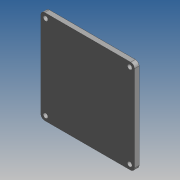
# Autodesk Inventor part: P035_FondBoitierv3
Saved by Autodesk Inventor 2021.3 (Build 253353000, 353)
## iProperties
Created: 2021-11-26
Part Number: P035_FondBoitierv3
Material: Générique
Document SubType Name: Modeling
Designer: gabri
Density: 1 g/cm^3
Appearance: Par défaut
Author: gabri
Autodesk Inventor part; units mm, degrees
ref_plane "YZ Plane" through (0, 0, 0) normal (1, 0, 0) x (0, 1, 0)
ref_plane "XZ Plane" through (0, 0, 0) normal (0, 1, 0) x (-1, 0, 0)
ref_plane "XY Plane" through (0, 0, 0) normal (0, 0, 1) x (1, 0, 0)
sketch "Sketch2" plane through (0, 0, 0) normal (0, 1, 0) x (-1, 0, 0)
  line L0 (-46, -50) -> (46, -50)
  line L1 (50, -46) -> (50, 46)
  line L2 (46, 50) -> (-46, 50)
  line L3 (-50, 46) -> (-50, -46)
  line L4 (-50, -50) -> (50, 50) construction
  line L5 (50, -50) -> (-50, 50) construction
  arc A0 (50, 46) -> (46, 50) centre (46, 46) ccw
  arc A1 (-46, 50) -> (-50, 46) centre (-46, 46) ccw
  arc A2 (-50, -46) -> (-46, -50) centre (-46, -46) ccw
  arc A3 (46, -50) -> (50, -46) centre (46, -46) ccw
  point P0 (0, 0)
  dimension "d0" = 100
  dimension "d1" = 100
  dimension "d4" = 4
  dimension "d5" = 4
  constraints: 12 end point, 8 point on circle, 8 point on line, 8 tangent, 4 centre point, 2 equal radius, 2 midpoint, 2 parallel, 1 horizontal, 1 perpendicular
  measures "d0" distance of L5.end L4.end
  measures "d1" distance between parallel lines of L0 L2
  measures "d4" radius of A0
  measures "d5" radius of A1
extrude "Extrusion1" add sketch "Sketch2" along normal blind 5
sketch "Sketch3" plane through (0, 0, 0) normal (0, -1, 0) x (1, 0, 0)
  arc A0 (-50, -46) -> (-46, -50) centre (-46, -46) ccw construction
  line L0 (46, -50) -> (-46, -50) construction
  arc A1 (46, -50) -> (50, -46) centre (46, -46) ccw construction
  line L1 (50, 46) -> (50, -46) construction
  arc A2 (50, 46) -> (46, 50) centre (46, 46) ccw construction
  line L2 (-46, 50) -> (46, 50) construction
  arc A3 (-46, 50) -> (-50, 46) centre (-46, 46) ccw construction
  line L3 (-50, -46) -> (-50, 46) construction
  point P0 (0, 0)
  point P1 (-45, 45)
  point P2 (45, 45)
  point P3 (-45, -45)
  point P4 (45, -45)
  dimension "d13" = 5
  dimension "d14" = 5
  dimension "d17" = 90
  dimension "d20" = 90
  constraints: 1 horizontal, 1 vertical, 3 other
  measures "d13" distance from line of L2 point (-45, 45)
  measures "d14" distance from line of L3 point (-45, 45)
  measures "d17" distance of point (-45, 45) point (45, 45)
  measures "d20" distance of point (-45, 45) point (-45, -45)
hole "Hole1" at (-45, 0, 45) at (45, 0, 45) at (45, 0, -45) at (-45, 0, -45) direction (0, 1, 0) diameter 5 depth 14.2 tip angle 118
sketch "Sketch4" plane through (0, 5, 0) normal (0, 1, 0) x (1, 0, 0)
  circle A0 centre (45, 45) radius 2.5 construction
  circle A1 centre (-45, -45) radius 2.5 construction
  circle A2 centre (45, -45) radius 2.5 construction
  circle A3 centre (-45, 45) radius 2.5 construction
  arc A4 (-46, 50) -> (-50, 46) centre (-46, 46) ccw construction
  line L0 (-50, 46) -> (-50, -46) construction
  arc A5 (-50, -46) -> (-46, -50) centre (-46, -46) ccw construction
  line L1 (-46, -50) -> (46, -50) construction
  arc A6 (46, -50) -> (50, -46) centre (46, -46) ccw construction
  line L2 (50, -46) -> (50, 46) construction
  arc A7 (50, 46) -> (46, 50) centre (46, 46) ccw construction
  line L3 (46, 50) -> (-46, 50) construction
  arc A8 (44.6333, -39.5122) -> (39.5122, -44.6333) centre (45, -45) ccw
  arc A9 (45.9545, -41.6327) -> (41.6327, -45.9545) centre (45, -45) ccw
  line L4 (39.7085, -48.5) -> (-39.7085, -48.5)
  line L5 (48.5, -39.7085) -> (48.5, 39.7085)
  line L6 (46.5, -37.5167) -> (46.5, 37.5167)
  line L7 (0, -72.209) -> (0, 64.6676) construction
  line L8 (107.9328, 0) -> (-102.5907, 0) construction
  line L9 (37.5167, -46.5) -> (-37.5167, -46.5)
  arc A10 (-39.5122, -44.6333) -> (-44.6333, -39.5122) centre (-45, -45) ccw
  arc A11 (-41.6327, -45.9545) -> (-45.9545, -41.6327) centre (-45, -45) ccw
  line L10 (-48.5, -39.7085) -> (-48.5, 39.7085)
  line L11 (-46.5, 37.5167) -> (-46.5, -37.5167)
  arc A12 (41.6327, 45.9545) -> (45.9545, 41.6327) centre (45, 45) ccw
  arc A13 (39.5122, 44.6333) -> (44.6333, 39.5122) centre (45, 45) ccw
  line L12 (39.7085, 48.5) -> (-39.7085, 48.5)
  line L13 (37.5167, 46.5) -> (-37.5167, 46.5)
  line L14 (46, 50) -> (-46, 50) construction
  arc A14 (-44.6333, 39.5122) -> (-39.5122, 44.6333) centre (-45, 45) ccw
  arc A15 (-45.9545, 41.6327) -> (-41.6327, 45.9545) centre (-45, 45) ccw
  arc A16 (39.7085, -48.5) -> (41.6327, -45.9545) centre (39.7085, -46.5) ccw
  arc A17 (37.5167, -46.5) -> (39.5122, -44.6333) centre (37.5167, -44.5) ccw
  arc A18 (45.9545, -41.6327) -> (48.5, -39.7085) centre (46.5, -39.7085) ccw
  arc A19 (44.6333, -39.5122) -> (46.5, -37.5167) centre (44.5, -37.5167) ccw
  arc A20 (-41.6327, -45.9545) -> (-39.7085, -48.5) centre (-39.7085, -46.5) ccw
  arc A21 (-39.5122, -44.6333) -> (-37.5167, -46.5) centre (-37.5167, -44.5) ccw
  arc A22 (-48.5, -39.7085) -> (-45.9545, -41.6327) centre (-46.5, -39.7085) ccw
  arc A23 (-46.5, -37.5167) -> (-44.6333, -39.5122) centre (-44.5, -37.5167) ccw
  arc A24 (-44.6333, 39.5122) -> (-46.5, 37.5167) centre (-44.5, 37.5167) ccw
  arc A25 (-45.9545, 41.6327) -> (-48.5, 39.7085) centre (-46.5, 39.7085) ccw
  arc A26 (-39.7085, 48.5) -> (-41.6327, 45.9545) centre (-39.7085, 46.5) ccw
  arc A27 (-37.5167, 46.5) -> (-39.5122, 44.6333) centre (-37.5167, 44.5) ccw
  arc A28 (41.6327, 45.9545) -> (39.7085, 48.5) centre (39.7085, 46.5) ccw
  arc A29 (39.5122, 44.6333) -> (37.5167, 46.5) centre (37.5167, 44.5) ccw
  arc A30 (48.5, 39.7085) -> (45.9545, 41.6327) centre (46.5, 39.7085) ccw
  arc A31 (46.5, 37.5167) -> (44.6333, 39.5122) centre (44.5, 37.5167) ccw
  point P0 (0, 0)
  point P1 (45, -48.5)
  point P2 (39.7085, -46.5)
  point P3 (48.5, -45)
  point P4 (48.5, 45)
  point P5 (46.5, -39.7085)
  point P6 (46.5, 39.7085)
  point P7 (-45, -48.5)
  point P8 (-48.5, -45)
  point P9 (-46.5, 39.7085)
  point P10 (-46.5, -39.7085)
  point P11 (45, 48.5)
  point P12 (-45, 48.5)
  point P13 (39.7085, 46.5)
  point P14 (-39.7085, 46.5)
  point P15 (-48.5, 45)
  dimension "d23" = 5.5
  dimension "d24" = 3.5
  dimension "d25" = 1.5
  dimension "d27" = 1.5
  dimension "d28" = 2
  dimension "d31" = 5.5
  dimension "d32" = 3.5
  dimension "d33" = 2
  dimension "d34" = 1.5
  dimension "d35" = 2
  dimension "d36" = 5.5
  dimension "d37" = 3.5
  dimension "d38" = 1.5
  dimension "d39" = 2
  dimension "d41" = 5.5
  dimension "d42" = 3.5
  dimension "d43" = 2
  dimension "d44" = 2
  dimension "d45" = 2
  constraints: 64 point on circle, 32 tangent, 24 centre point, 20 end point, 16 point on line, 13 equal radius, 8 coincident, 6 parallel, 4 horizontal, 1 vertical
  measures "d23" radius of A8
  measures "d24" radius of A9
  measures "d25" distance between parallel lines of L1 L4
  measures "d27" distance between parallel lines of L2 L5
  measures "d28" distance between parallel lines of L5 L6
  measures "d31" radius of A10
  measures "d32" radius of A11
  measures "d33" distance between parallel lines of L9 L4
  measures "d34" distance between parallel lines of L0 L10
  measures "d35" distance between parallel lines of L10 L11
  measures "d36" radius of A13
  measures "d37" radius of A12
  measures "d38" distance between parallel lines of L3 L12
  measures "d39" distance between parallel lines of L12 L13
  measures "d41" radius of A14
  measures "d42" radius of A15
  measures "d43" radius of A16
  measures "d44" radius of A17
  measures "d45" radius of A20
extrude "Extrusion2" cut sketch "Sketch4" against normal blind 2
body "Solid1"
